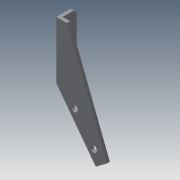
# Autodesk Inventor part: pracka_leva1
Saved by Autodesk Inventor 2013 (Build 170138000, 138)
## iProperties
Created: 2013-02-02
Part Number: pracka_leva1
Material: Generic
Document SubType Name: Modeling
Designer: idle-rug
Density: 1 g/cm^3
Author: idle-rug
Autodesk Inventor part; units mm, degrees
ref_plane "YZ Plane" through (0, 0, 0) normal (1, 0, 0) x (0, 1, 0)
ref_plane "XZ Plane" through (0, 0, 0) normal (0, 1, 0) x (-1, 0, 0)
ref_plane "XY Plane" through (0, 0, 0) normal (0, 0, 1) x (1, 0, 0)
sketch "Sketch2" plane through (0, 0, 0) normal (0, 1, 0) x (-1, 0, 0)
  line L0 (0.0014, 0.0009) -> (-14.9986, -19.9991)
  line L1 (0.0014, 0.0009) -> (-7.9986, 0.0009)
  line L2 (0.0014, 37.0009) -> (0.0014, 0.0009)
  line L3 (0.0014, 37.0009) -> (-7.9986, 0.0009)
  line L4 (-7.9986, 0.0009) -> (-20.8467, -17.1298)
  circle A0 centre (-8.4986, -5.9991) radius 1.5
  circle A1 centre (-17.4986, -17.9991) radius 1.5
  line L5 (-21.0986, -22.7991) -> (-18.5386, -24.7191)
  line L6 (-20.8467, -17.1298) -> (-23.6586, -20.8791)
  line L7 (-23.6586, -20.8791) -> (-18.5386, -24.7191)
  line L8 (-18.5386, -24.7191) -> (-14.9986, -19.9991)
  point P0 (0, 0)
  dimension "d4" = 3
  dimension "d5" = 3
  constraints: 18 end point, 2 centre point, 1 collinear, 1 horizontal, 1 parallel, 1 perpendicular
  measures "d4" diameter of A0
  measures "d5" diameter of A1
extrude "Extrusion1" add sketch "Sketch2" along normal blind 2
sketch "Sketch3" plane through (0, 2, 0) normal (0, 1, 0) x (1, 0, 0)
  line L0 (-0.0014, -0.0009) -> (-0.0014, -37.0009) projected
  line L1 (-0.0014, -37.0009) -> (7.9986, -0.0009) projected
  line L2 (7.9986, -0.0009) -> (23.6586, 20.8791) projected
  line L3 (-0.0014, -37.0009) -> (9.9986, -37.0009)
  line L4 (9.9986, -37.0009) -> (23.6586, 20.8791)
  point P0 (0, 0)
  dimension "d8" = 10
  constraints: 4 end point, 1 perpendicular
  measures "d8" distance of L0.end L3.end
extrude "Extrusion2" add sketch "Sketch3" against normal blind 2
sketch "Sketch4" plane through (0, 2, 0) normal (0, 1, 0) x (1, 0, 0)
  line L0 (-0.0014, -37.0009) -> (9.9986, -37.0009) projected
  line L1 (9.9986, -37.0009) -> (23.6586, 20.8791) projected
  line L2 (4.9986, -37.0009) -> (23.6586, 20.8791)
  line L3 (4.9986, -37.0009) -> (9.9986, -37.0009)
  line L4 (9.9986, -37.0009) -> (23.6586, 20.8791)
  point P0 (0, 0)
  dimension "d13" = 5
  constraints: 6 end point, 2 collinear, 1 midpoint
  measures "d13" distance of L0.start L2.start
extrude "Extrusion3" cut sketch "Sketch4" against normal blind 2
sketch "Sketch6" plane through (0, 2, 0) normal (0, 1, 0) x (1, 0, 0)
  line L0 (-0.0014, -37.0009) -> (4.9986, -37.0009) projected
  line L1 (0, 0) -> (2, 0)
  line L2 (2, 0) -> (2, -37.0009)
  line L3 (-0.0014, -37.0009) -> (2, -37.0009)
  line L4 (-0.0014, -37.0009) -> (0, 0)
  dimension "d16" = 2
  constraints: 8 end point, 1 collinear, 1 parallel, 1 perpendicular, 1 point on line
  measures "d16" distance of L1.start L1.end
extrude "Extrusion4" add sketch "Sketch6" along normal blind 6
sketch "Sketch9" plane through (0, 0, 0) normal (0, -1, 0) x (1, 0, 0)
  line L0 (23.6586, -20.8791) -> (4.9986, 37.0009) projected
  line L1 (4.9986, 37.0009) -> (-0.0014, 37.0009) projected
  line L2 (-0.0014, 0.0009) -> (-0.0014, 37.0009) projected
  line L3 (-0.0014, 37.0009) -> (-0.0014, 27.0012)
  line L4 (-0.0014, 27.0012) -> (4.9986, 27.0012)
  line L5 (4.9986, 27.0012) -> (23.6586, -20.8791)
  line L6 (23.6586, -20.8791) -> (4.9986, 37.0009)
  line L7 (-0.0014, 37.0009) -> (4.9986, 37.0009)
  point P0 (0, 0)
  constraints: 10 end point, 2 collinear, 1 perpendicular, 1 point on line
extrude "Extrusion5" cut sketch "Sketch9" against normal blind 10
sketch "Sketch10" plane through (0, 2, 0) normal (0, 1, 0) x (1, 0, 0)
  line L0 (-0.0014, -27.0012) -> (-0.001, -27.0012) projected
  line L1 (-0.001, -27.0012) -> (0, 0) projected
  line L2 (0, 0) -> (2, 0) projected
  line L3 (2, 0) -> (2, -27.0012) projected
  line L4 (2, -27.0012) -> (4.9986, -27.0012) projected
  line L5 (4.9986, -27.0012) -> (23.6586, 20.8791) projected
  line L6 (23.6586, 20.8791) -> (18.5386, 24.7191) projected
  line L7 (18.5386, 24.7191) -> (-0.0014, -0.0009) projected
  line L8 (-0.0014, -0.0009) -> (-0.0014, -27.0012) projected
  circle A0 centre (8.4986, 5.9991) radius 1.5 projected
  circle A1 centre (17.4986, 17.9991) radius 1.5 projected
extrude "Extrusion6" cut sketch "Sketch10" against normal blind 0.5
sketch "Sketch11" plane through (2, 8, 27.0012) normal (1, 0, 0) x (0, 0, -1)
  line L0 (0, -6.5) -> (0, 0) projected
  line L1 (0, -6.5) -> (27.0012, -6.5) projected
  line L2 (27.0012, 0) -> (27.0012, -6.5) projected
  line L3 (0, 0) -> (27.0012, 0) projected
  point P0 (27.0012, -8)
extrude "Extrusion7" cut sketch "Sketch11" against normal blind 0.5
fillet "Fillet1" radius 2 1 edges at (0.7495, 8, 27.0012)
fillet "Fillet2" radius 2 1 edges at (0.75, 8, 0)
body "Solid1"
